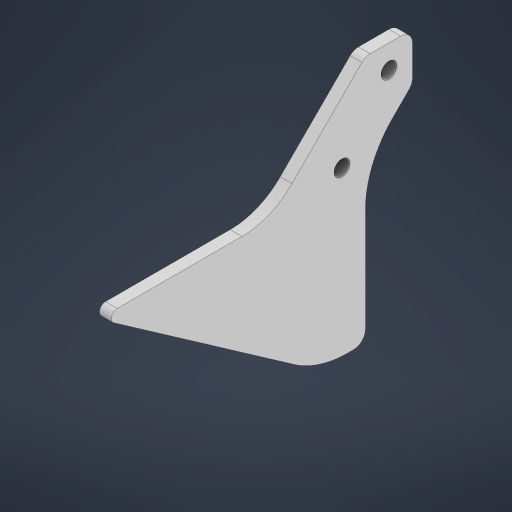
# Autodesk Inventor part: flip out sleds
Saved by Autodesk Inventor 2024 (Build 280153000, 153)
## iProperties
Created: 2024-03-28
Part Number: flip out sleds
Material: Generic
Document SubType Name: Modeling
Designer: Andrew
Density: 1 g/cm^3
Appearance: Default
Author: Andrew
Autodesk Inventor part; units mm, degrees
ref_plane "YZ Plane" through (0, 0, 0) normal (1, 0, 0) x (0, 1, 0)
ref_plane "XZ Plane" through (0, 0, 0) normal (0, 1, 0) x (-1, 0, 0)
ref_plane "XY Plane" through (0, 0, 0) normal (0, 0, 1) x (1, 0, 0)
sketch "Sketch1" plane through (0, 0, 0) normal (1, 0, 0) x (0, 1, 0)
  line L0 (0, 0) -> (0, -12.7)
  line L1 (0, 0) -> (41.5212, 59.2984)
  line L2 (41.5212, 59.2984) -> (41.5212, -12.7)
  line L3 (41.5212, -12.7) -> (0, -12.7)
  line L4 (41.5212, 2.0806) -> (41.5212, -12.7)
  line L5 (41.5212, -12.7) -> (66.9212, -12.7)
  line L6 (41.5212, 8.3226) -> (41.5212, -12.7)
  line L7 (41.5212, 0) -> (66.9212, 0)
  line L8 (66.9212, 0) -> (66.9212, -12.7)
  line L9 (66.9212, -12.7) -> (41.5212, -12.7)
  line L10 (41.5212, -12.7) -> (41.5212, 0)
  line L11 (41.5212, -6.35) -> (44.0612, -6.35)
  circle A0 centre (44.0612, -6.35) radius 2.1082
  line L12 (66.9212, -12.7) -> (54.2212, -12.7)
  line L13 (54.2212, -12.7) -> (54.2212, -25.4)
  line L14 (54.2212, -25.4) -> (66.9212, -25.4)
  line L15 (66.9212, -25.4) -> (66.9212, -12.7)
  circle A1 centre (60.5712, -19.05) radius 2.1082
  line L16 (54.2212, 0) -> (66.9212, -12.7)
  line L17 (54.2212, -25.4) -> (41.5212, -12.7)
  line L18 (54.2212, 0) -> (41.5212, 12.7)
  point P0 (41.5212, 8.3226)
  point P1 (41.5212, 0)
  point P2 (41.5212, -12.7)
  dimension "d0" = 12.7
  dimension "d1" = 72.39
  dimension "d3" = 145
  dimension "d20" = 2.54
  dimension "d22" = 4.2164
  dimension "d23" = 12.7
  dimension "d24" = 12.7
  dimension "d25" = 25.4
  dimension "d26" = 25.4
  dimension "d27" = 4.2164
  dimension "d30" = 45
  constraints: 38 end point, 5 parallel, 4 horizontal, 3 perpendicular, 2 centre point, 2 midpoint, 2 point on line, 2 vertical, 1 coincident
  measures "d0" distance of L0.start L0.end
  measures "d1" distance of L0.start L1.end
  measures "d3" angle of L0 L1
  measures "d20" distance of L11.start L11.end
  measures "d22" diameter of A0
  measures "d23" distance of L12.end L13.end
  measures "d24" distance of L13.end L14.end
  measures "d25" distance of L7.start L7.end
  measures "d26" distance of L2.end L5.end
  measures "d27" diameter of A1
  measures "d30" angle of L7 L18
extrude "Extrusion1" add sketch "Sketch1" along normal blind 3.175 contours L1 L2 L3 L0 | L2 L7 L16 L5 | L5 L13 L17 | L18 L7 L2 | L5 L15 L14 L13
fillet "Fillet1" radius 1.5875 1 edges at (1.5875, 41.5212, 59.2984)
fillet "Fillet7" radius 19.05 1 edges at (1.5875, 41.5212, 12.7)
fillet "Fillet8" radius 25.4 1 edges at (1.5875, 41.5212, -12.7)
fillet "Fillet9" radius 3.175 4 edges at (1.5875, 54.2212, -25.4) (1.5875, 66.9212, -25.4) (1.5875, 66.9212, -12.7) (1.5875, 0, -12.7)
fillet "Fillet10" radius 25.4 1 edges at (1.5875, 0, 0)
body "Solid1"
